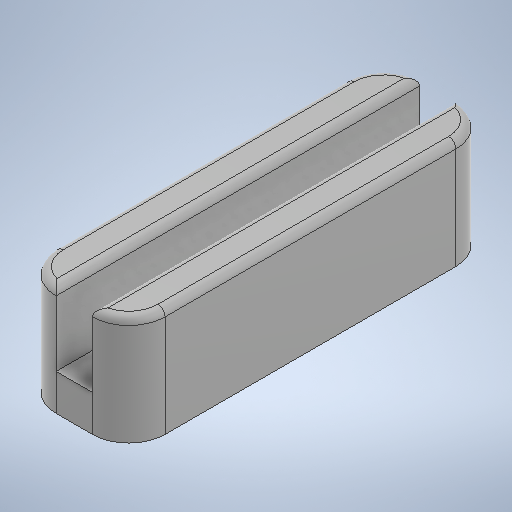
# Autodesk Inventor part: TSU_Middle_Top_Clamp
Saved by Autodesk Inventor 2025.2 (Build 292293000, 293)
## iProperties
Created: 2025-01-07
Part Number: TSU_Middle_Top_Clamp
Material: Generic
Document SubType Name: Modeling
Designer: Matt Tidd
Density: 1 g/cm^3
Appearance: Default
Author: Matt Tidd
Autodesk Inventor part; units mm, degrees
ref_plane "YZ Plane" through (0, 0, 0) normal (1, 0, 0) x (0, 1, 0)
ref_plane "XZ Plane" through (0, 0, 0) normal (0, 1, 0) x (-1, 0, 0)
ref_plane "XY Plane" through (0, 0, 0) normal (0, 0, 1) x (1, 0, 0)
sketch "Sketch1" plane through (0, 0, 0) normal (0, 1, 0) x (-1, 0, 0)
  line L0 (0, 0) -> (30, 0)
  line L1 (30, 0) -> (30, -100)
  line L2 (30, -100) -> (0, -100)
  line L3 (0, -100) -> (0, 0)
  dimension "d0" = 30
  dimension "d1" = 100
  constraints: 8 end point, 2 parallel, 1 horizontal, 1 perpendicular
  measures "d0" distance of L1.end L2.end
  measures "d1" distance of L0.end L1.end
extrude "Extrusion1" add sketch "Sketch1" along normal blind 10
sketch "Sketch2" plane through (0, 10, 0) normal (0, 1, 0) x (1, 0, 0)
  line L0 (-30, 0) -> (0, 0) projected
  line L1 (0, 0) -> (-10, 0)
  line L2 (-10, 0) -> (-10, 100)
  line L3 (-10, 100) -> (0, 100)
  line L4 (0, 100) -> (0, 0)
  line L5 (-30, 0) -> (-20, 0)
  line L6 (-20, 0) -> (-20, 100)
  line L7 (-20, 100) -> (-30, 100)
  line L8 (-30, 100) -> (-30, 0)
  dimension "d4" = 10
  dimension "d5" = 100
  dimension "d6" = 10
  dimension "d7" = 100
  constraints: 16 end point, 4 parallel, 2 horizontal, 2 perpendicular
  measures "d4" distance of L2.end L3.end
  measures "d5" distance of L1.end L2.end
  measures "d6" distance of L7.end L6.end
  measures "d7" distance of L6.end L5.end
extrude "Extrusion2" add sketch "Sketch2" along normal blind 20
sketch "Sketch3" plane through (-20, 10, 0) normal (1, 0, 0) x (0, 0, -1)
  line L0 (100, 20) -> (0, 20) construction
  line L1 (50, 20) -> (50, 0) construction
  line L2 (0, 0) -> (100, 0) construction
  point P0 (0, -10)
  constraints: 2 end point, 2 midpoint
fillet "Fillet1" radius 10 4 edges at (0, 15, 0) (-30, 15, 0) (0, 15, -100) (-30, 15, -100)
fillet "Fillet2" radius 2 8 edges at (-27.0711, 30, -2.9289) (-27.0711, 30, -97.0711) (-30, 30, -50) (-20, 30, -50) (-10, 30, -50) (-2.9289, 30, -97.0711) (-2.9289, 30, -2.9289) (0, 30, -50)
body "Solid1"
